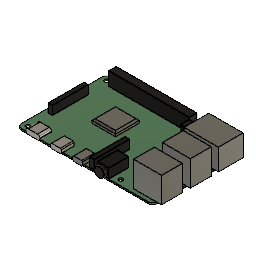
dummy (Autodesk Fusion 360 design; units mm, degrees)
Autodesk Fusion 360 part; units mm, degrees
sketch "Skizze4" plane through (0, 0, 0) normal (0, 0, 1) x (1, 0, 0)
  line L0 (52.4999, -25) -> (52.4999, 24.6406)
  line L1 (-32.5, 24.5) -> (-32.5, -25.0196)
  line L2 (49.5215, 28) -> (-29.5, 28)
  line L3 (-32.5, 25) -> (-32.5, 24.5)
  line L4 (49.4999, -28) -> (-29.5, -28)
  line L5 (-32.5, -25) -> (-32.5, -25.0196)
  circle A0 centre (29, 24.5) radius 1.3
  circle A1 centre (29, -24.5) radius 1.3
  circle A2 centre (-29, -24.5) radius 1.3
  circle A3 centre (-29, 24.5) radius 1.3
  arc A4 (-29.5, 28) -> (-32.5, 25) centre (-29.5, 25) ccw
  arc A5 (-32.5, -25) -> (-29.5, -28) centre (-29.5, -25) ccw
  arc A6 (49.4999, -28) -> (52.4999, -25) centre (49.4999, -25) ccw
  arc A7 (52.4999, 24.6406) -> (49.5215, 28) centre (49.5215, 25) ccw
  line L6 (-29, 24.5) -> (29, -24.5) construction
  line L7 (29, 24.5) -> (-29, -24.5) construction
  line L8 (-29, 24.5) -> (-29, -24.5) construction
  line L9 (-29, -24.5) -> (29, -24.5) construction
  line L10 (29, -24.5) -> (29, 24.5) construction
  line L11 (-29, 24.5) -> (29, 24.5) construction
  point P0 (-32.5, 28)
  dimension "d3" = 85
  dimension "d6" = 3.5
  dimension "d11" = 2.6
  dimension "d17" = 3
  dimension "d57" = 49
  dimension "d58" = 58
  dimension "d61" = 56
  dimension "d62" = 3.5
  dimension "d63" = 3.5
  constraint parallel L0 L1
  constraint horizontal L2
  constraint vertical L3
  constraint horizontal L4
  constraint vertical L5
  constraint coincident P0 L2
  constraint coincident P0 L3
  constraint tangent L2 A4
  constraint tangent L3 A4
  constraint tangent L4 A5
  constraint tangent L5 A5
  constraint tangent L4 A6
  constraint equal A5 A6
  constraint tangent L2 A7
  constraint equal A5 A7
  constraint equal A4 A5
  constraint equal A1 A2
  constraint equal A2 A3
  constraint equal A0 A3
  constraint coincident L0.end A7.start
  constraint coincident A3.centre L6.start
  constraint coincident A1.centre L6.end
  constraint coincident A0.centre L7.start
  constraint coincident A2.centre L7.end
  constraint midpoint L6 origin
  constraint coincident L0.start A6.end
  constraint midpoint L7 origin
  constraint vertical L0
  constraint horizontal L11
  constraint vertical L10
  constraint tangent L0 A6
  measures "d3" distance of L0.end L1.start
  measures "d6" distance of L1.start P0
  measures "d11" diameter of A2
  measures "d17" radius of A4
  measures "d57" distance of A2.centre A3.centre
  measures "d58" distance of A0.centre A3.centre
  measures "d61" distance of L2 L4
  measures "d62" distance of L1 A3.centre
  measures "d63" distance of L2 A3.centre
extrude "Extrusion7" add sketch "Skizze4" along normal blind 1 makes body 1
copy_body "Körper->Berechn3" bodies 1 removing the originals makes body 2 in component "Baseplate"
sketch "Skizze9" plane through (0, 0, 1) normal (0, 0, 1) x (1, 0, 0)
  arc A0 (52.4999, 24.6406) -> (49.5215, 28) centre (49.5215, 25) ccw
  line L0 (52.4999, -25) -> (52.4999, 24.6406) construction
  line L1 (49.5215, 28) -> (-29.5, 28) construction
  arc A1 (49.4999, -28) -> (52.4999, -25) centre (49.4999, -25) ccw construction
  line L2 (49.4999, -28) -> (-29.5, -28) construction
  circle A2 centre (29, -24.5) radius 1.3
  arc A3 (-29.5, 28) -> (-32.5, 25) centre (-29.5, 25) ccw construction
  line L3 (-32.5, 24.5) -> (-32.5, -25.0196) construction
  arc A4 (-32.5, -25) -> (-29.5, -28) centre (-29.5, -25) ccw construction
  circle A5 centre (29, 24.5) radius 1.3
  circle A6 centre (-29, 24.5) radius 1.3
  circle A7 centre (-29, -24.5) radius 1.3
  line L4 (-32.5, 25) -> (-32.5, 24.5) construction
  circle A8 centre (29, -24.5) radius 1.3
  circle A9 centre (29, 24.5) radius 1.3
  circle A10 centre (-29, -24.5) radius 1.3
  circle A11 centre (-29, 24.5) radius 1.3
  arc A12 (49.4999, -28) -> (52.4999, -25) centre (49.4999, -25) ccw
  line L5 (52.4999, -25) -> (52.4999, 24.6406)
  arc A13 (52.4999, 24.6406) -> (49.5215, 28) centre (49.5215, 25) ccw
  line L6 (49.5215, 28) -> (-29.5, 28)
  arc A14 (-29.5, 28) -> (-32.5, 25) centre (-29.5, 25) ccw
  line L7 (-32.5, 25) -> (-32.5, -25)
  arc A15 (-32.5, -25) -> (-29.5, -28) centre (-29.5, -25) ccw
  line L8 (-29.5, -28) -> (49.4999, -28)
  line L9 (-16.9308, -29.1603) -> (-25.6692, -29.1603)
  line L10 (-25.6692, -29.1603) -> (-25.6692, -21.785)
  line L11 (-25.6692, -21.785) -> (-16.9308, -21.785)
  line L12 (-16.9308, -21.785) -> (-16.9308, -29.1603)
  line L13 (-16.9308, -29.1603) -> (-25.6692, -21.785) construction
  line L14 (-25.6692, -29.1603) -> (-16.9308, -21.785) construction
  line L15 (-3.25, -29.5) -> (-9.75, -29.5)
  line L16 (-9.75, -29.5) -> (-9.75, -21.5)
  line L17 (-9.75, -21.5) -> (-3.25, -21.5)
  line L18 (-3.25, -21.5) -> (-3.25, -29.5)
  line L19 (-3.25, -29.5) -> (-9.75, -21.5) construction
  line L20 (-9.75, -29.5) -> (-3.25, -21.5) construction
  line L21 (10, -29.5) -> (4, -29.5)
  line L22 (4, -29.5) -> (4, -21.5)
  line L23 (4, -21.5) -> (10, -21.5)
  line L24 (10, -21.5) -> (10, -29.5)
  line L25 (10, -29.5) -> (4, -21.5) construction
  line L26 (4, -29.5) -> (10, -21.5) construction
  line L27 (18, -28) -> (25, -28)
  line L28 (25, -28) -> (25, -15.5)
  line L29 (25, -15.5) -> (18, -15.5)
  line L30 (18, -15.5) -> (18, -28)
  line L31 (18, -28) -> (25, -15.5) construction
  line L32 (25, -28) -> (18, -15.5) construction
  line L33 (55.4999, -25.5) -> (37.9999, -25.5)
  line L34 (37.9999, -25.5) -> (37.9999, -12.5)
  line L35 (37.9999, -12.5) -> (55.4999, -12.5)
  line L36 (55.4999, -12.5) -> (55.4999, -25.5)
  line L37 (55.4999, -25.5) -> (37.9999, -12.5) construction
  line L38 (37.9999, -25.5) -> (55.4999, -12.5) construction
  line L39 (55.4999, -7.5) -> (37.9999, -7.5)
  line L40 (37.9999, -7.5) -> (37.9999, 5.5)
  line L41 (37.9999, 5.5) -> (55.4999, 5.5)
  line L42 (55.4999, 5.5) -> (55.4999, -7.5)
  line L43 (55.4999, -7.5) -> (37.9999, 5.5) construction
  line L44 (37.9999, -7.5) -> (55.4999, 5.5) construction
  line L45 (55.4999, 10) -> (33.9999, 10)
  line L46 (33.9999, 10) -> (33.9999, 25.5)
  line L47 (33.9999, 25.5) -> (55.4999, 25.5)
  line L48 (55.4999, 25.5) -> (55.4999, 10)
  line L49 (55.4999, 10) -> (33.9999, 25.5) construction
  line L50 (33.9999, 10) -> (55.4999, 25.5) construction
  line L51 (25.2404, 22.1337) -> (-25.2404, 22.1337)
  line L52 (-25.2404, 22.1337) -> (-25.2404, 26.8663)
  line L53 (-25.2404, 26.8663) -> (25.2404, 26.8663)
  line L54 (25.2404, 26.8663) -> (25.2404, 22.1337)
  line L55 (25.2404, 22.1337) -> (-25.2404, 26.8663) construction
  line L56 (-25.2404, 22.1337) -> (25.2404, 26.8663) construction
  line L57 (-29, 24.5) -> (29, 24.5) construction
  line L58 (-27.0854, -11.1703) -> (-29.7923, -11.1703)
  line L59 (-29.7923, -11.1703) -> (-29.7923, 11.318)
  line L60 (-29.7923, 11.318) -> (-27.0854, 11.318)
  line L61 (-27.0854, 11.318) -> (-27.0854, -11.1703)
  line L62 (-27.0854, -11.1703) -> (-29.7923, 11.318) construction
  line L63 (-29.7923, -11.1703) -> (-27.0854, 11.318) construction
  line L64 (4.2156, -2.9834) -> (-10.5748, -2.9834)
  line L65 (-10.5748, -2.9834) -> (-10.5748, 11.807)
  line L66 (-10.5748, 11.807) -> (4.2156, 11.807)
  line L67 (4.2156, 11.807) -> (4.2156, -2.9834)
  line L68 (4.2156, -2.9834) -> (-10.5748, 11.807) construction
  line L69 (-10.5748, -2.9834) -> (4.2156, 11.807) construction
  line L70 (15.4032, -27.5854) -> (12.5968, -27.5854)
  line L71 (12.5968, -27.5854) -> (12.5968, -5.4146)
  line L72 (12.5968, -5.4146) -> (15.4032, -5.4146)
  line L73 (15.4032, -5.4146) -> (15.4032, -27.5854)
  line L74 (15.4032, -27.5854) -> (12.5968, -5.4146) construction
  line L75 (12.5968, -27.5854) -> (15.4032, -5.4146) construction
  line L76 (-16.614, -8.6626) -> (-24.2715, -8.6626)
  line L77 (-24.2715, -8.6626) -> (-24.2715, -6.5905)
  line L78 (-24.2715, -6.5905) -> (-16.614, -6.5905)
  line L79 (-16.614, -6.5905) -> (-16.614, -8.6626)
  line L80 (-16.614, -8.6626) -> (-24.2715, -6.5905) construction
  line L81 (-24.2715, -8.6626) -> (-16.614, -6.5905) construction
  line L82 (-3.25, -29.5) -> (4, -29.5) construction
  line L83 (-3.25, -21.5) -> (4, -21.5) construction
  line L84 (55.4999, -12.5) -> (55.4999, -7.5) construction
  line L85 (55.4999, 5.5) -> (55.4999, 10) construction
  line L86 (31.6, 15.6523) -> (26.4, 15.6523)
  line L87 (26.4, 15.6523) -> (26.4, 20.8523)
  line L88 (26.4, 20.8523) -> (31.6, 20.8523)
  line L89 (31.6, 20.8523) -> (31.6, 15.6523)
  line L90 (31.6, 15.6523) -> (26.4, 20.8523) construction
  line L91 (26.4, 15.6523) -> (31.6, 20.8523) construction
  point P0 (-21.3, -25.4727)
  point P1 (-6.5, -25.5)
  point P2 (7, -25.5)
  point P3 (21.5, -21.75)
  point P4 (46.7499, -19)
  point P5 (46.7499, -1)
  point P6 (44.7499, 17.75)
  point P7 (0, 24.5)
  point P8 (-28.4388, 0.0739)
  point P9 (-3.1796, 4.4118)
  point P10 (14, -16.5)
  point P11 (-20.4428, -7.6266)
  point P12 (29, 18.2523)
  dimension "d66" = 9
  dimension "d67" = 27
  dimension "d68" = 45.75
  dimension "d69" = 29
  dimension "d70" = 7.7
  dimension "d71" = 14.8
  dimension "d72" = 13.5
  dimension "d73" = 6.5
  dimension "d74" = 6
  dimension "d75" = 8
  dimension "d76" = 17.5
  dimension "d77" = 13
  dimension "d78" = 1.5
  dimension "d79" = 12.5
  dimension "d80" = 7
  dimension "d82" = 7
  dimension "d84" = 7.5
  dimension "d85" = 3
  dimension "d86" = 21.5
  dimension "d87" = 15.5
  dimension "d88" = 5.2
  dimension "d89" = 5.2
  dimension "d90" = 11.5
  dimension "d91" = 17.5
  dimension "d92" = 13
  constraint perpendicular L9 L10
  constraint parallel L9 L11
  constraint parallel L10 L12
  constraint horizontal L9
  constraint coincident L13 P0
  constraint coincident L14 P0
  constraint perpendicular L15 L16
  constraint parallel L15 L17
  constraint parallel L16 L18
  constraint horizontal L15
  constraint coincident L19 P1
  constraint coincident L20 P1
  constraint perpendicular L21 L22
  constraint parallel L21 L23
  constraint parallel L22 L24
  constraint horizontal L21
  constraint coincident L25 P2
  constraint coincident L26 P2
  constraint perpendicular L27 L28
  constraint parallel L27 L29
  constraint parallel L28 L30
  constraint horizontal L27
  constraint coincident L31 P3
  constraint coincident L32 P3
  constraint coincident L2 L27.end
  constraint perpendicular L33 L34
  constraint parallel L33 L35
  constraint parallel L34 L36
  constraint horizontal L33
  constraint coincident L37 P4
  constraint coincident L38 P4
  constraint perpendicular L39 L40
  constraint parallel L39 L41
  constraint parallel L40 L42
  constraint horizontal L39
  constraint coincident L43 P5
  constraint coincident L44 P5
  constraint perpendicular L45 L46
  constraint parallel L45 L47
  constraint parallel L46 L48
  constraint horizontal L45
  constraint coincident L49 P6
  constraint coincident L50 P6
  constraint perpendicular L51 L52
  constraint parallel L51 L53
  constraint parallel L52 L54
  constraint horizontal L51
  constraint coincident L55 P7
  constraint coincident L56 P7
  constraint coincident A6.centre A11.centre
  constraint coincident A5.centre A9.centre
  constraint coincident P7 L57
  constraint perpendicular L58 L59
  constraint parallel L58 L60
  constraint parallel L59 L61
  constraint horizontal L58
  constraint coincident L62 P8
  constraint coincident L63 P8
  constraint perpendicular L64 L65
  constraint parallel L64 L66
  constraint parallel L65 L67
  constraint horizontal L64
  constraint coincident L68 P9
  constraint coincident L69 P9
  constraint perpendicular L70 L71
  constraint parallel L70 L72
  constraint parallel L71 L73
  constraint horizontal L70
  constraint coincident L74 P10
  constraint coincident L75 P10
  constraint perpendicular L76 L77
  constraint parallel L76 L78
  constraint parallel L77 L79
  constraint horizontal L76
  constraint coincident L80 P11
  constraint coincident L81 P11
  constraint horizontal L82
  constraint horizontal L83
  constraint perpendicular L41 L85
  constraint vertical L84
  constraint perpendicular L86 L87
  constraint parallel L86 L88
  constraint parallel L87 L89
  constraint horizontal L86
  constraint coincident L90 P12
  constraint coincident L91 P12
  measures "d66" distance of L2 P4
  measures "d67" distance of L2 P5
  measures "d68" distance of L2 P6
  measures "d69" distance of P7 A6.centre
  measures "d70" horizontal distance of A7.centre P0
  measures "d71" horizontal distance of P0 P1
  measures "d72" distance of P1 P2
  measures "d73" distance of L16 L18
  measures "d74" distance of L22 L24
  measures "d75" distance of L15 L17
  measures "d76" distance of L34.end L35.end
  measures "d77" distance of L33.start L35.end
  measures "d78" distance of L2 L21
  measures "d79" distance of L27.end L28.end
  measures "d80" distance of L28.end L29.end
  measures "d82" horizontal distance of P2 P10
  measures "d84" horizontal distance of P3 P10
  measures "d85" distance of L0 L84
  measures "d86" distance of L46.end L47.end
  measures "d87" distance of L45.end L46.end
  measures "d88" distance of L86.end L87.end
  measures "d89" distance of L87.end L88.end
  measures "d90" distance of L2 P10
  measures "d91" distance of L39.start L39.end
  measures "d92" distance of L39.start L41.end
extrude "Extrusion8" add sketch "Skizze9" along normal blind 3.2 separate body contours L8 L10 L11 L12 | L8 L9 L10 L12 makes body 3
extrude "Extrusion9" add sketch "Skizze9" along normal blind 3 separate body contours L8 L16 L17 L18 | L8 L15 L16 L18 | L8 L21 L22 L24 | L8 L22 L23 L24 makes body 4 at (-7.5833, -26.8333, 1) makes body 5 at (6, -24.1667, 1)
extrude "Extrusion10" add sketch "Skizze9" along normal blind 5.5 separate body contours L58 L59 L60 L61 | L70 L71 L72 L73 makes body 6 at (12.5968, -20.1951, 2.8333) makes body 7 at (-29.7923, -3.6742, 2.8333)
extrude "Extrusion11" add sketch "Skizze9" along normal blind 6 separate body contours L8 L27 L28 L29 L30 makes body 8
extrude "Extrusion12" add sketch "Skizze9" along normal blind 16 separate body contours L5 L39 L41 L42 | L5 L39 L40 L41 | A12 L5 L33 L35 L36 | A12 L5 L33 L34 L35 makes body 9 at (43.8332, -12.5, 6.3333) makes body 10 at (43.8332, 5.5, 6.3333)
extrude "Extrusion13" add sketch "Skizze9" along normal blind 13.5 separate body contours A0 L5 A13 L45 L46 L47 | A0 L5 A13 L45 L47 L48 makes body 11
extrude "Extrusion14" add sketch "Skizze9" along normal blind 8.5 separate body contours L51 L52 L53 L54 | L86 L87 L88 L89 makes body 12 at (8.4135, 22.1337, 3.8333) makes body 13 at (26.4, 17.3856, 3.8333)
extrude "Extrusion15" add sketch "Skizze9" along normal blind 2.4 separate body contours L64 L65 L66 L67 makes body 14
sketch "Skizze10" plane through (0, -28, 0) normal (0, -1, 0) x (1, 0, 0)
  line L0 (18, 1) -> (25, 1)
  line L1 (25, 1) -> (25, 7)
  line L2 (25, 7) -> (18, 7)
  line L3 (18, 7) -> (18, 1)
  circle A0 centre (21.5, 4) radius 3
  line L4 (18, 7) -> (25, 1) construction
  line L5 (25, 7) -> (18, 1) construction
  constraint tangent L0 A0
  constraint coincident L2.end L3.start
  constraint coincident L0.end L1.start
  constraint coincident L1.end L2.start
  constraint coincident L0.start L3.end
  constraint coincident A0.centre L5
  constraint coincident A0.centre L4
extrude "Extrusion16" add sketch "Skizze10" along normal blind 2.5 contours A0 bodies 8
fillet "Abrundung1" radius 1.5 4 edges at (-25.6692, -25.4727, 4.2) (-25.6692, -25.4727, 1) (-16.9308, -25.4727, 4.2) (-16.9308, -25.4727, 1) on bodies 3
chamfer "Fase4" distance 1 angle 45 4 edges at (-10.5748, 4.4118, 3.4) (-3.1796, -2.9834, 3.4) (-3.1796, 11.807, 3.4) (4.2156, 4.4118, 3.4) on bodies 14
fillet "Abrundung2" radius 0.5 8 edges at (-9.75, -25.5, 4) (-3.25, -25.5, 4) (-9.75, -25.5, 1) (-3.25, -25.5, 1) (4, -25.5, 1) (4, -25.5, 4) (10, -25.5, 4) (10, -25.5, 1) on bodies 4 5
copy_body "Körper->Berechn4" bodies 3 removing the originals makes body 15 in component "Power USB C"
copy_body "Körper->Berechn5" bodies 5 removing the originals makes body 16 in component "Micro HDMI 2"
copy_body "Körper->Berechn6" bodies 8 removing the originals makes body 17 in component "3.5 mm Audio"
copy_body "Körper->Berechn7" bodies 4 removing the originals makes body 18 in component "Micro HDMI 1"
copy_body "Körper->Berechn8" bodies 9 removing the originals makes body 19 in component "USB 2.0"
copy_body "Körper->Berechn9" bodies 7 removing the originals makes body 20 in component "Display"
copy_body "Körper->Berechn10" bodies 14 removing the originals makes body 21 in component "Processor"
copy_body "Körper->Berechn11" bodies 11 removing the originals makes body 22 in component "Ethernet "
copy_body "Körper->Berechn12" bodies 6 removing the originals makes body 23 in component "Kamera"
copy_body "Körper->Berechn13" bodies 12 removing the originals makes body 24 in component "GPIO 40"
copy_body "Körper->Berechn14" bodies 10 removing the originals makes body 25 in component "USB 3.0"
copy_body "Körper->Berechn15" bodies 13 removing the originals makes body 26 in component "PoE"
sketch "Skizze11" plane through (0, 0, 0) normal (0, 0, -1) x (1, 0, 0)
  circle A0 centre (29, 24.5) radius 1.3
  circle A1 centre (-29, 24.5) radius 1.3
  circle A2 centre (-29, -24.5) radius 1.3
  circle A3 centre (29, -24.5) radius 1.3
  arc A4 (52.4999, 25) -> (49.4999, 28) centre (49.4999, 25) ccw
  line L0 (49.4999, 28) -> (-29.5, 28)
  arc A5 (-29.5, 28) -> (-32.5, 25) centre (-29.5, 25) ccw
  line L1 (-32.5, 25) -> (-32.5, -25)
  arc A6 (-32.5, -25) -> (-29.5, -28) centre (-29.5, -25) ccw
  line L2 (-29.5, -28) -> (49.5215, -28)
  arc A7 (49.5215, -28) -> (52.4999, -24.6406) centre (49.5215, -25) ccw
  line L3 (52.4999, -24.6406) -> (52.4999, 25)
  line L4 (-29, 24.5) -> (-29, -24.5) construction
  line L5 (-23, 5.5) -> (-35, 5.5)
  line L6 (-35, 5.5) -> (-35, -5.5)
  line L7 (-35, -5.5) -> (-23, -5.5)
  line L8 (-23, -5.5) -> (-23, 5.5)
  line L9 (-23, 5.5) -> (-35, -5.5) construction
  line L10 (-35, 5.5) -> (-23, -5.5) construction
  point P0 (-29, 0)
  dimension "d114" = 11
  dimension "d115" = 12
  constraint coincident A1.centre L4.start
  constraint coincident A2.centre L4.end
  constraint perpendicular L5 L6
  constraint parallel L5 L7
  constraint parallel L6 L8
  constraint horizontal L5
  constraint coincident L9 P0
  constraint coincident L10 P0
  constraint midpoint L4 P0
  measures "d114" distance of L5.end L6.end
  measures "d115" distance of L6.end L7.end
extrude "Extrusion1" add sketch "Skizze11" along normal blind 1.2 separate body contours L1 L5 L7 L8 | L1 L5 L6 L7 makes body 27 in component "Baseplate"
fillet "Abrundung1'" radius 0.6 2 edges at (-35, 5.5, -0.6) (-35, -5.5, -0.6) on bodies 27 in component "Baseplate"
component "Baseplate" placed x (1, 0, 0) y (0, 1, 0) z (0, 0, 1) at (0, 0, 0)
component "Power USB C" placed x (1, 0, 0) y (0, 1, 0) z (0, 0, 1) at (0, 0, 0)
component "Micro HDMI 2" placed x (1, 0, 0) y (0, 1, 0) z (0, 0, 1) at (0, 0, 0)
component "3.5 mm Audio" placed x (1, 0, 0) y (0, 1, 0) z (0, 0, 1) at (0, 0, 0)
component "Micro HDMI 1" placed x (1, 0, 0) y (0, 1, 0) z (0, 0, 1) at (0, 0, 0)
component "USB 2.0" placed x (1, 0, 0) y (0, 1, 0) z (0, 0, 1) at (0, 0, 0)
component "Display" placed x (1, 0, 0) y (0, 1, 0) z (0, 0, 1) at (0, 0, 0)
component "Processor" placed x (1, 0, 0) y (0, 1, 0) z (0, 0, 1) at (0, 0, 0)
component "Ethernet " placed x (1, 0, 0) y (0, 1, 0) z (0, 0, 1) at (0, 0, 0)
component "Kamera" placed x (1, 0, 0) y (0, 1, 0) z (0, 0, 1) at (0, 0, 0)
component "GPIO 40" placed x (1, 0, 0) y (0, 1, 0) z (0, 0, 1) at (0, 0, 0)
component "USB 3.0" placed x (1, 0, 0) y (0, 1, 0) z (0, 0, 1) at (0, 0, 0)
component "PoE" placed x (1, 0, 0) y (0, 1, 0) z (0, 0, 1) at (0, 0, 0)
equation "d91 = d76"
equation "d92 = d77"
named bodies: "Power USB C", "Micro HDMI 1", "Micro HDMI 2", "Kamera", "Display", "3.5 mm Audio", "USB 2.0", "USB 3.0", "Ethernet", "GPIO 40", "PoE", "Processor"
